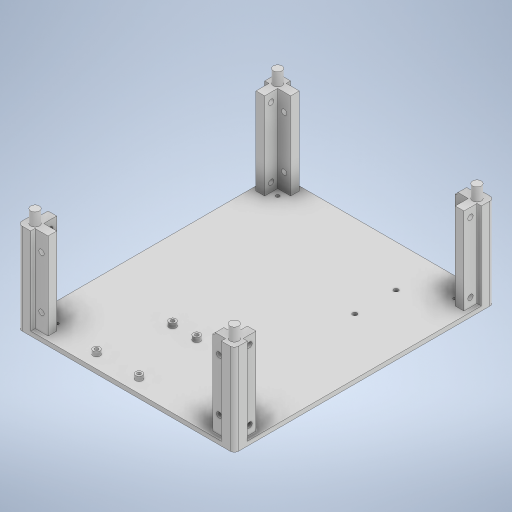
# Autodesk Inventor part: Bottom
Saved by Autodesk Inventor 2024 (Build 280153000, 153)
## iProperties
Created: 2026-03-15
Part Number: Bottom
Material: Generic
Document SubType Name: Modeling
Designer: HP
Density: 1 g/cm^3
Appearance: Default
Author: HP
Autodesk Inventor part; units mm, degrees
ref_plane "YZ Plane" through (0, 0, 0) normal (1, 0, 0) x (0, 1, 0)
ref_plane "XZ Plane" through (0, 0, 0) normal (0, 1, 0) x (-1, 0, 0)
ref_plane "XY Plane" through (0, 0, 0) normal (0, 0, 1) x (1, 0, 0)
sketch "Sketch1" plane through (0, 0, 0) normal (0, 1, 0) x (-1, 0, 0)
  line L0 (0, 0) -> (0, 150)
  line L1 (0, 150) -> (0, -150)
  line L2 (0, -150) -> (125, -150)
  line L3 (125, -150) -> (125, 150)
  line L4 (125, 150) -> (-125, 150)
  line L5 (-125, 150) -> (-125, -150)
  line L6 (-125, -150) -> (0, -150)
  dimension "d0" = 150
  dimension "d1" = 300
  dimension "d2" = 125
  dimension "d3" = 300
  dimension "d4" = 250
  dimension "d5" = 300
  constraints: 14 end point, 3 perpendicular, 2 point on line, 1 vertical
  measures "d0" distance of L0.start L0.end
  measures "d1" distance of L0.end L1.end
  measures "d2" distance of L1.end L2.end
  measures "d3" distance of L2.end L3.end
  measures "d4" distance of L3.end L4.end
  measures "d5" distance of L4.end L5.end
extrude "Extrusion1" add sketch "Sketch1" along normal blind 5
fillet "Fillet1" radius 5 1 edges at (125, 2.5, 150)
fillet "Fillet2" radius 5 3 edges at (125, 2.5, -150) (-125, 2.5, -150) (-125, 2.5, 150)
sketch "Sketch2" plane through (0, 5, 0) normal (0, 1, 0) x (1, 0, 0)
  line L0 (120, 150) -> (-120, 150) projected
  line L1 (-120, 150) -> (-110, 150)
  line L2 (-110, 150) -> (-110, 145)
  line L3 (-110, 145) -> (-101.6, 145)
  arc A0 (-120, 150) -> (-125, 145) centre (-120, 145) ccw projected
  line L4 (-125, 145) -> (-125, 135)
  line L5 (-125, 145) -> (-125, -145) projected
  line L6 (-125, 135) -> (-120, 135)
  line L7 (-120, 135) -> (-120, 120)
  line L8 (-110, 145) -> (-95, 145)
  arc A1 (-120, 150) -> (-125, 145) centre (-120, 145) ccw
  line L9 (125, -145) -> (125, 145) projected
  line L10 (125, 0) -> (-125, 0)
  line L11 (0, 150) -> (0, -150)
  line L12 (-120, -150) -> (120, -150) projected
  line L13 (-95, 145) -> (-95, 135)
  line L14 (-120, 120) -> (-110, 120)
  line L15 (-95, 135) -> (-110, 135)
  line L16 (-110, 135) -> (-110, 120)
  line L17 (-120, -150) -> (-110, -150)
  line L18 (-110, -150) -> (-110, -145)
  line L19 (-125, -145) -> (-125, -135)
  line L20 (-125, -135) -> (-120, -135)
  line L21 (-120, -135) -> (-120, -120)
  line L22 (-110, -145) -> (-95, -145)
  arc A2 (-125, -145) -> (-120, -150) centre (-120, -145) ccw
  line L23 (-95, -145) -> (-95, -135)
  line L24 (-120, -120) -> (-110, -120)
  line L25 (-95, -135) -> (-110, -135)
  line L26 (-110, -135) -> (-110, -120)
  line L27 (-120, 150) -> (120, 150)
  line L28 (110, 150) -> (110, 145)
  line L29 (125, 145) -> (125, -145)
  line L30 (125, 135) -> (120, 135)
  line L31 (120, 135) -> (120, 120)
  line L32 (110, 145) -> (95, 145)
  arc A3 (125, 145) -> (120, 150) centre (120, 145) ccw
  line L33 (120, -150) -> (-120, -150)
  line L34 (95, 145) -> (95, 135)
  line L35 (120, 120) -> (110, 120)
  line L36 (95, 135) -> (110, 135)
  line L37 (110, 135) -> (110, 120)
  line L38 (95, -135) -> (110, -135)
  line L39 (95, -145) -> (95, -135)
  line L40 (110, -150) -> (110, -145)
  line L41 (120, -150) -> (110, -150)
  arc A4 (120, -150) -> (125, -145) centre (120, -145) ccw
  line L42 (125, -135) -> (120, -135)
  line L43 (120, -135) -> (120, -120)
  line L44 (120, -120) -> (110, -120)
  line L45 (110, -135) -> (110, -120)
  line L46 (110, -145) -> (95, -145)
  point P0 (0, 0)
  point P1 (-101.6, -145)
  dimension "d10" = 10
  dimension "d11" = 5
  dimension "d12" = 10
  dimension "d13" = 5
  dimension "d14" = 15
  dimension "d15" = 15
  dimension "d17" = 10
  dimension "d18" = 10
  constraints: 86 end point, 35 symmetric about line, 8 point on circle, 5 point on line, 4 centre point, 4 midpoint, 4 perpendicular, 3 horizontal, 2 tangent, 1 vertical, 3 other
  measures "d10" distance of L0.end L1.end
  measures "d11" distance of L1.end L2.end
  measures "d12" distance of L4.start L4.end
  measures "d13" distance of L4.end L6.end
  measures "d14" distance of L6.end L7.end
  measures "d15" distance of L2.end L8.end
  measures "d17" distance of L8.end L13.end
  measures "d18" distance of L7.end L14.end
extrude "Extrusion2" add sketch "Sketch2" along normal blind 100 contours A3 L9 L30 L31 L35 L37 L36 L34 L32 L28 L0 | L2 L3 L8 L13 L15 L16 L14 L7 L6 L4 A0 L0 | L9 A4 L12 L40 L46 L39 L38 L45 L44 L43 L42 | L20 L21 L24 L26 L25 L23 L22 L18 L12 A2 L5
sketch "Sketch3" plane through (0, 105, 0) normal (0, 1, 0) x (1, 0, 0)
  line L0 (120, 150) -> (-120, 150) projected
  line L1 (0, 150) -> (0, -150)
  line L2 (-120, -150) -> (120, -150) projected
  line L3 (0, 0) -> (125, 0)
  line L4 (125, -135) -> (125, 135) projected
  line L5 (0, 0) -> (-125, 0)
  line L6 (-125, 135) -> (-125, -135) projected
  line L7 (95, 145) -> (95, 135) projected
  line L8 (95, 145) -> (95, 140)
  line L9 (95, 140) -> (125, 140)
  line L10 (110, 120) -> (120, 120) projected
  line L11 (120, 120) -> (115, 120)
  line L12 (115, 120) -> (115, 140)
  circle A0 centre (115, 140) radius 5
  circle A1 centre (115, -140) radius 5
  circle A2 centre (-115, 140) radius 5
  circle A3 centre (-115, -140) radius 5
  constraints: 14 end point, 6 midpoint, 4 centre point, 3 symmetric about line, 1 coincident, 1 horizontal, 1 perpendicular, 1 point on line, 3 other
extrude "Extrusion3" add sketch "Sketch3" along normal blind 15
sketch "Sketch4" plane through (-120, 5, -135) normal (-1, 0, 0) x (0, 0, 1)
  line L0 (15, 100) -> (0, 100) projected
  line L1 (0, 100) -> (7.5, 100)
  line L2 (7.5, 100) -> (7.5, 90)
  line L3 (7.5, 90) -> (7.5, 10)
  point P0 (135, -5)
  dimension "d23" = 7.5
  dimension "d24" = 10
  dimension "d25" = 80
  constraints: 6 end point, 1 midpoint, 1 perpendicular, 1 point on line
  measures "d23" distance of L0.end L1.end
  measures "d24" distance of L1.end L2.end
  measures "d25" distance of L2.end L3.end
hole "Hole1" at (-120, 95, -127.5) at (-120, 15, -127.5) direction (1, 0, 0) diameter 6 end through all
sketch "Sketch5" plane through (-120, 5, 120) normal (-1, 0, 0) x (0, 0, 1)
  line L0 (15, 100) -> (0, 100) projected
  line L1 (0, 100) -> (7.5, 100)
  line L2 (7.5, 100) -> (7.5, 90)
  line L3 (7.5, 90) -> (7.5, 10)
  point P0 (-120, -5)
  dimension "d35" = 10
  dimension "d36" = 80
  constraints: 6 end point, 1 midpoint, 1 point on line, 1 vertical
  measures "d35" distance of L1.end L2.end
  measures "d36" distance of L2.end L3.end
hole "Hole2" at (-120, 95, 127.5) at (-120, 15, 127.5) direction (1, 0, 0) diameter 6 end through all
sketch "Sketch6" plane through (-110, 5, 145) normal (0, 0, 1) x (1, 0, 0)
  line L0 (0, 0) -> (0, 100) projected
  line L1 (0, 100) -> (7.5, 100)
  line L2 (15, 100) -> (0, 100) projected
  line L3 (7.5, 100) -> (7.5, 80)
  line L4 (7.5, 80) -> (7.5, 20)
  line L5 (220, 0) -> (220, 100) projected
  line L6 (220, 100) -> (212.5, 100)
  line L7 (205, 100) -> (220, 100) projected
  line L8 (212.5, 100) -> (212.5, 80)
  line L9 (212.5, 80) -> (212.5, 20)
  point P0 (110, -5)
  dimension "d44" = 20
  dimension "d45" = 60
  constraints: 12 end point, 2 midpoint, 2 point on line, 2 vertical
  measures "d44" distance of L1.end L3.end
  measures "d45" distance of L3.end L4.end
hole "Hole3" at (-102.5, 85, 145) at (-102.5, 25, 145) direction (0, 0, -1) diameter 6 end through all
sketch "Sketch7" plane through (95, 5, 145) normal (0, 0, 1) x (1, 0, 0)
  line L0 (0, 100) -> (7.5, 100)
  line L1 (0, 100) -> (15, 100) projected
  line L2 (7.5, 100) -> (7.5, 80)
  line L3 (7.5, 80) -> (7.5, 20)
  point P0 (-95, -5)
  dimension "d53" = 20
  dimension "d54" = 60
  constraints: 6 end point, 1 midpoint, 1 perpendicular, 1 point on line
  measures "d53" distance of L0.end L2.end
  measures "d54" distance of L2.end L3.end
hole "Hole4" at (95, 105, 145) at (102.5, 85, 145) at (102.5, 25, 145) direction (0, 0, -1) diameter 6 end through all
sketch "Sketch8" plane through (0, 5, 0) normal (0, 1, 0) x (1, 0, 0)
  line L0 (-120, -150) -> (120, -150) projected
  line L1 (0, -150) -> (0, -135)
  line L2 (0, -135) -> (80.9625, -135)
  line L3 (80.9625, -135) -> (-82.55, -135)
  line L4 (0, -135) -> (-49, -135)
  line L5 (-49, -135) -> (-49, -62.9)
  line L6 (0, -135) -> (0, -62.9)
  line L7 (-49, -62.9) -> (-33.376, -62.9)
  line L8 (-33.376, -62.9) -> (-5.467, -62.9)
  line L9 (-5.467, -62.9) -> (0, -62.9)
  circle A0 centre (0, -135) radius 2
  circle A1 centre (-49, -135) radius 2
  circle A2 centre (-5.467, -62.9) radius 2
  circle A3 centre (-33.376, -62.9) radius 2
  circle A4 centre (-5.467, -62.9) radius 4
  circle A5 centre (-33.376, -62.9) radius 4
  circle A6 centre (-49, -135) radius 4
  circle A7 centre (0, -135) radius 4
  point P0 (0, 0)
  dimension "d62" = 15
  dimension "d63" = 49
  dimension "d64" = 72.1
  dimension "d67" = 15.624
  dimension "d68" = 27.909
  dimension "d69" = 4
  dimension "d70" = 4
  dimension "d71" = 4
  dimension "d72" = 4
  dimension "d73" = 8
  dimension "d74" = 8
  dimension "d75" = 8
  dimension "d76" = 8
  constraints: 18 end point, 8 centre point, 8 coincident, 3 point on line, 2 perpendicular, 2 vertical, 1 collinear, 1 horizontal, 1 midpoint
  measures "d62" distance of L1.start L1.end
  measures "d63" distance of L1.end L4.end
  measures "d64" distance of L4.end L5.end
  measures "d67" distance of L5.end L7.end
  measures "d68" distance of L7.end L8.end
  measures "d69" diameter of A0
  measures "d70" diameter of A1
  measures "d71" diameter of A2
  measures "d72" diameter of A3
  measures "d73" diameter of A4
  measures "d74" diameter of A5
  measures "d75" diameter of A6
  measures "d76" diameter of A7
extrude "Extrusion4" add sketch "Sketch8" along normal blind 5 contours A7 L3 A0 L1 | L1 A0 L2 A7 | A7 L6 A0 L3 | L2 A0 L6 A7 | A6 L3 A1 | L3 A1 L5 A6 | L5 A1 L3 A6 | A4 L8 A2 L9 | L9 A2 L8 A4 | A5 L8 A3 L7 | L7 A3 L8 A5
sketch "Sketch9" plane through (-5.467, 5, 62.9) normal (0, 1, 0) x (1, 0, 0)
  circle A0 centre (0, 0) radius 2 projected
  circle A1 centre (0, 0) radius 2
  circle A2 centre (5.467, -72.1) radius 4 projected
  circle A3 centre (5.467, -72.1) radius 2
  circle A4 centre (-43.533, -72.1) radius 2 projected
  circle A5 centre (-43.533, -72.1) radius 2
  circle A6 centre (-27.909, 0) radius 2 projected
  circle A7 centre (-27.909, 0) radius 2
  point P0 (5.467, 62.9)
  dimension "d79" = 4
  dimension "d80" = 4
  dimension "d81" = 4
  dimension "d82" = 4
  constraints: 4 centre point, 4 coincident
  measures "d79" diameter of A1
  measures "d80" diameter of A3
  measures "d81" diameter of A5
  measures "d82" diameter of A7
extrude "Extrusion5" cut sketch "Sketch9" against normal blind 10 contours A0 | A3 | A4 | A6
sketch "Sketch10" plane through (0, 5, 0) normal (0, 1, 0) x (1, 0, 0)
  line L0 (0, 0) -> (0, 101.6)
  line L1 (0, 101.6) -> (60, 101.6)
  line L2 (60, 101.6) -> (60, 54.1)
  circle A0 centre (60, 101.6) radius 2.5
  circle A1 centre (60, 54.1) radius 2.5
  dimension "d85" = 60
  dimension "d86" = 47.5
  dimension "d87" = 5
  dimension "d88" = 5
  constraints: 6 end point, 2 centre point, 2 coincident, 1 horizontal, 1 perpendicular, 1 vertical
  measures "d85" distance of L0.end L1.end
  measures "d86" distance of L1.end L2.end
  measures "d87" diameter of A0
  measures "d88" diameter of A1
extrude "Extrusion6" cut sketch "Sketch10" against normal blind 10
sketch "Sketch11" plane through (0, 5, 0) normal (0, 1, 0) x (1, 0, 0)
  line L0 (-110, 120) -> (-110, 135) projected
  line L1 (-110, 135) -> (-110, 127.5)
  line L2 (-110, 135) -> (-95, 135) projected
  line L3 (-95, 135) -> (-95, 127.5)
  line L4 (-95, 127.5) -> (-110, 127.5)
  line L5 (-95, 127.5) -> (-102.5, 127.5)
  line L6 (125, -135) -> (125, 135) projected
  line L7 (125, 0) -> (-125, 0)
  line L8 (-125, 135) -> (-125, -135) projected
  line L9 (110, 150) -> (-110, 150) projected
  line L10 (0, 150) -> (0, -150)
  line L11 (-120, -150) -> (120, -150) projected
  circle A0 centre (-102.5, 127.5) radius 2
  circle A1 centre (-102.5, -127.5) radius 2
  circle A2 centre (102.5, 127.5) radius 2
  circle A3 centre (102.5, -127.5) radius 2
  point P0 (0, 0)
  dimension "d91" = 4
  constraints: 12 end point, 6 midpoint, 4 centre point, 3 symmetric about line, 1 coincident, 1 perpendicular, 1 vertical, 3 other
  measures "d91" diameter of A0
extrude "Extrusion7" cut sketch "Sketch11" against normal blind 15 contours A0 L4 | L4 A0 | A1 | A2 | A3
body "Solid1"
